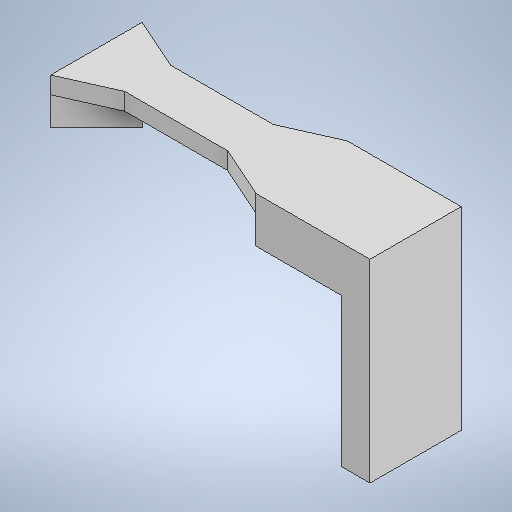
# Autodesk Inventor part: Connecting pt.1
Saved by Autodesk Inventor 2025.2 (Build 292293000, 293)
## iProperties
Created: 2025-04-14
Part Number: Connecting pt.1
Material: Generic
Document SubType Name: Modeling
Designer: 1khanhan2
Density: 1 g/cm^3
Appearance: Default
Author: 1khanhan2
Autodesk Inventor part; units mm, degrees
ref_plane "YZ Plane" through (0, 0, 0) normal (1, 0, 0) x (0, 1, 0)
ref_plane "XZ Plane" through (0, 0, 0) normal (0, 1, 0) x (-1, 0, 0)
ref_plane "XY Plane" through (0, 0, 0) normal (0, 0, 1) x (1, 0, 0)
sketch "Sketch1" plane through (0, 0, 0) normal (0, 1, 0) x (-1, 0, 0)
  line L0 (0, 0) -> (0, -16)
  line L1 (8, -8) -> (0, 0)
  line L2 (8, -8) -> (0, -16)
  line L3 (0, 0) -> (-20, 0)
  line L4 (-20, 0) -> (-20, -16)
  line L5 (-20, -16) -> (0, -16)
  dimension "d0" = 16
  dimension "d2" = 20
  constraints: 12 end point, 2 perpendicular, 1 horizontal, 1 vertical
  measures "d0" distance of L0.start L0.end
  measures "d2" distance of L0.start L3.end
extrude "Extrusion1" add sketch "Sketch1" along normal blind 5
sketch "Sketch2" plane through (0, 0, 0) normal (0, -1, 0) x (1, 0, 0)
  line L0 (20, -16) -> (0, -16) projected
  line L1 (20, -16) -> (15, -16)
  line L2 (15, -16) -> (15, 0)
  line L3 (0, 0) -> (20, 0) projected
  line L4 (20, 0) -> (20, -16) projected
  line L5 (20, 0) -> (20, -16)
  line L6 (20, -16) -> (18.5, -16)
  line L7 (15, -16) -> (15, -14.5)
  line L8 (15, -16) -> (16.5, -16)
  line L9 (16.5, -14.5) -> (18.5, -14.5)
  line L10 (18.5, -14.5) -> (18.5, -1.5)
  line L11 (18.5, -1.5) -> (16.5, -1.5)
  line L12 (16.5, -1.5) -> (16.5, -14.5)
  dimension "d5" = 5
  dimension "d8" = 1.5
  dimension "d9" = 1.5
  dimension "d11" = 13
  constraints: 20 end point, 5 point on line, 3 perpendicular, 1 collinear, 1 vertical
  measures "d5" distance of L0.start L1.end
  measures "d8" distance of L0.start L6.end
  measures "d9" distance of L6.end L9.end
  measures "d11" distance of L9.end L10.end
extrude "Extrusion2" add sketch "Sketch2" along normal blind 26
extrude "Extrusion3" add sketch "Sketch2" along normal blind 27 contours L12 L11 L10 L9
sketch "Sketch3" plane through (0, 5, 0) normal (0, 1, 0) x (1, 0, 0)
  line L0 (0, 0) -> (20, 0) projected
  line L1 (20, 16) -> (0, 16) projected
  line L2 (0, 0) -> (0, 16)
  line L3 (0, 16) -> (-8, 8) projected
  line L4 (0, 16) -> (-8, 8)
  line L5 (-8, 8) -> (0, 0)
  line L6 (0, 0) -> (-36, 0)
  line L7 (-36, 0) -> (-28, 8)
  line L8 (-28, 8) -> (-36, 16)
  line L9 (-36, 16) -> (0, 16)
  line L10 (-36, 16) -> (-36, 0)
  dimension "d14" = 36
  dimension "d15" = 45
  constraints: 16 end point, 2 equal length, 2 perpendicular, 1 horizontal, 1 vertical
  measures "d14" distance of L0.start L6.end
  measures "d15" angle of L6 L7
extrude "Extrusion4" add sketch "Sketch3" against normal blind 5 contours L10 L8 L7
sketch "Sketch4" plane through (0, 5, 0) normal (0, 1, 0) x (1, 0, 0)
  line L0 (-28, 8) -> (-36, 0) projected
  line L1 (20, 16) -> (20, 0) projected
  line L2 (-36, 0) -> (20, 0)
  line L3 (20, 0) -> (20, 16)
  line L4 (20, 16) -> (-36, 16)
  line L5 (-36, 16) -> (-36, 0)
  line L6 (-36, 8) -> (20, 8)
  line L7 (-28, 8) -> (-8, 8)
  line L8 (-36, 16) -> (-18, 8)
  line L9 (-36, 0) -> (-18, 8)
  line L10 (0, 0) -> (-18, 8)
  line L11 (0, 16) -> (-8, 8) projected
  line L12 (0, 16) -> (-18, 8)
  line L13 (-27, 12) -> (-9, 12)
  line L14 (-27, 4) -> (-9, 4)
  constraints: 24 end point, 8 midpoint, 4 equal length, 1 horizontal, 1 perpendicular
extrude "Extrusion5" add sketch "Sketch4" along normal blind 3 contours L6 L9 L0 | L0 L5 L6 | L6 L5 L8 | L12 L11 L6 | L10 L14 L9 | L6 L1 L2 L10 | L8 L13 L12 | L11 L4 L1 L6
body "Solid1"
